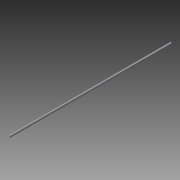
# Autodesk Inventor part: Pied
Saved by Autodesk Inventor 2015 SP1 (Build 190203100, 203)
## iProperties
Created: 2015-05-01
Part Number: Pied
Material: Générique
Document SubType Name: Modeling
Designer: Cyril
Density: 1 g/cm^3
Appearance: Par défaut
Author: Cyril
Autodesk Inventor part; units mm, degrees
ref_plane "YZ Plane" through (0, 0, 0) normal (1, 0, 0) x (0, 1, 0)
ref_plane "XZ Plane" through (0, 0, 0) normal (0, 1, 0) x (-1, 0, 0)
ref_plane "XY Plane" through (0, 0, 0) normal (0, 0, 1) x (1, 0, 0)
sketch "Sketch1" plane through (0, 0, 0) normal (0, 1, 0) x (-1, 0, 0)
  line L0 (10, 10) -> (-10, 10)
  line L1 (-10, 10) -> (-10, -10)
  line L2 (-10, -10) -> (10, -10)
  line L3 (10, -10) -> (10, 10)
  line L4 (10, 10) -> (-10, -10) construction
  line L5 (-10, 10) -> (10, -10) construction
  line L6 (8, 8) -> (-8, 8)
  line L7 (-8, 8) -> (-8, -8)
  line L8 (-8, -8) -> (8, -8)
  line L9 (8, -8) -> (8, 8)
  line L10 (8, 8) -> (-8, -8) construction
  line L11 (-8, 8) -> (8, -8) construction
  point P0 (0, 0)
  dimension "d0" = 20
  dimension "d1" = 20
  dimension "d2" = 2
  constraints: 24 end point, 4 midpoint, 4 parallel, 2 horizontal, 2 perpendicular, 1 point on line
  measures "d0" distance of L0.start L0.end
  measures "d1" distance of L2.end L0.start
  measures "d2" distance between parallel lines of L0 L6
extrude "Extrusion1" add sketch "Sketch1" along normal mid plane 2300
sketch "Sketch2" plane through (10, -1150, 10) normal (0, 0, 1) x (1, 0, 0)
  line L0 (0, 0) -> (-20, 20)
  line L1 (-20, 0) -> (-20, 2300) projected
  line L2 (-20, 0) -> (-20, 20)
  line L3 (-20, 0) -> (0, 0)
  line L4 (0, 0) -> (0, 2300) projected
  point P0 (-10, 1150)
  dimension "d5" = 45
  constraints: 6 end point, 2 point on line, 1 collinear, 1 perpendicular
  measures "d5" angle of L3 L0
extrude "Extrusion2" cut sketch "Sketch2" against normal through all
equation "\"d1\" = d0"
body "Solid1"
